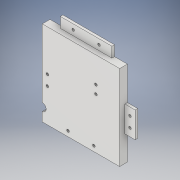
# Autodesk Inventor part: CP007
Saved by Autodesk Inventor 2017 SP1 (Build 210196100, 196)
## iProperties
Created: 2017-05-15
Part Number: CP007
Material: ABS Plastic
Document SubType Name: Modeling
Designer: zallen
Density: 1.06 g/cm^3
Appearance: Smooth - White
Mass: 391.263 g
Surface Area: 662.381 cm^2
Volume: 369.116 cm^3
Author: zallen
Autodesk Inventor part; units mm, degrees
ref_plane "YZ Plane" through (0, 0, 0) normal (1, 0, 0) x (0, 1, 0)
ref_plane "XZ Plane" through (0, 0, 0) normal (0, 1, 0) x (-1, 0, 0)
ref_plane "XY Plane" through (0, 0, 0) normal (0, 0, 1) x (1, 0, 0)
sketch "Sketch1" plane through (0, 0, 0) normal (0, 0, 1) x (1, 0, 0)
  line L0 (0, 0) -> (150, 0)
  line L1 (150, 0) -> (150, 164.5751)
  line L2 (150, 164.5751) -> (0, 164.5751)
  line L3 (0, 164.5751) -> (0, 0)
  dimension "d0" = 150
  dimension "d1" = 164.5751
  constraints: 8 end point, 2 parallel, 1 horizontal, 1 perpendicular
  measures "d0" distance of L2.end L1.end
  measures "d1" distance of L1.end L0.end
extrude "Extrusion1" add sketch "Sketch1" along normal blind 15
sketch "Sketch7" plane through (0, 0, 0) normal (0, 0, -1) x (-1, 0, 0)
  line L0 (-20, 50) -> (0, 50)
  line L1 (0, 50) -> (0, 100)
  line L2 (0, 100) -> (-20, 100)
  line L3 (-20, 100) -> (-20, 50)
  line L4 (0, 164.5751) -> (0, 0) projected
  dimension "d27" = 20
  dimension "d28" = 50
  dimension "d96" = 50
  constraints: 8 end point, 2 parallel, 1 horizontal, 1 perpendicular, 1 point on line
  measures "d27" distance of L2.end L1.end
  measures "d28" distance of L1.end L0.end
  measures "d96" distance of L0.end L4.end
extrude "Extrusion7" cut sketch "Sketch7" against normal blind 5
sketch "Sketch8" plane through (0, 0, 0) normal (0, 0, -1) x (-1, 0, 0)
  line L0 (-150, 164.5751) -> (0, 164.5751) projected
  line L1 (-25, 164.5751) -> (-125, 164.5751)
  line L2 (-125, 164.5751) -> (-125, 184.5751)
  line L3 (-125, 184.5751) -> (-25, 184.5751)
  line L4 (-25, 184.5751) -> (-25, 164.5751)
  point P0 (0, 0)
  dimension "d37" = 100
  dimension "d38" = 20
  dimension "d126" = 25
  constraints: 8 end point, 2 parallel, 1 horizontal, 1 perpendicular, 1 point on line
  measures "d37" distance of L2.end L3.end
  measures "d38" distance of L1.end L2.end
  measures "d126" distance from line of point (0, 0) L4
extrude "Extrusion8" add sketch "Sketch8" against normal blind 5
sketch "Sketch9" plane through (0, 0, 0) normal (0, 0, -1) x (-1, 0, 0)
  circle A0 centre (-50, 174.5751) radius 2.5
  circle A1 centre (-100, 174.5751) radius 2.5
  line L0 (-125, 184.5751) -> (-25, 184.5751) projected
  line L1 (0, 100) -> (0, 50) projected
  line L2 (0, 25) -> (20, 25) projected
  line L3 (20, 75) -> (0, 75) projected
  point P0 (0, 0)
  dimension "d44" = 5
  dimension "d45" = 5
  dimension "d46" = 10
  constraints: 2 centre point, 1 horizontal alignment
  measures "d44" diameter of A0
  measures "d45" diameter of A1
  measures "d46" distance from line of L0 A0.centre
extrude "Extrusion9" cut sketch "Sketch9" against normal through all
thread "Thread1" size "M5x0.8" class "6H" standard "ANSI Metric M Profile" full length
thread "Thread2" size "M5x0.8" class "6H" standard "ANSI Metric M Profile" full length
sketch "Sketch12" plane through (0, 0, 0) normal (0, 0, -1) x (-1, 0, 0)
  line L0 (0, 0) -> (-150, 0) projected
  line L1 (-25, 0) -> (-125, 0)
  line L2 (-125, 0) -> (-125, 20)
  line L3 (-125, 20) -> (-25, 20)
  line L4 (-25, 20) -> (-25, 0)
  dimension "d79" = 100
  dimension "d80" = 20
  dimension "d81" = 25
  constraints: 8 end point, 2 parallel, 1 horizontal, 1 perpendicular, 1 point on line
  measures "d79" distance of L2.end L3.end
  measures "d80" distance of L1.end L2.end
  measures "d81" distance from line of L0.start L4
extrude "Extrusion12" cut sketch "Sketch12" against normal blind 5
sketch "Sketch13" plane through (0, 0, 5) normal (0, 0, -1) x (-1, 0, 0)
  circle A0 centre (-50, 10) radius 2.5
  circle A1 centre (-100, 10) radius 2.5
  line L0 (-25, 20) -> (-25, 0) projected
  line L1 (-125, 0) -> (-125, 20) projected
  line L2 (-125, 20) -> (-25, 20) projected
  point P0 (0, 0)
  dimension "d84" = 5
  dimension "d85" = 5
  dimension "d86" = 25
  dimension "d87" = 25
  dimension "d88" = 10
  dimension "d89" = 10
  constraints: 2 centre point
  measures "d84" diameter of A0
  measures "d85" diameter of A1
  measures "d86" distance from line of A0.centre L0
  measures "d87" distance from line of L1 A1.centre
  measures "d88" distance from line of L2 A0.centre
  measures "d89" distance from line of L2 A1.centre
extrude "Extrusion13" cut sketch "Sketch13" against normal through all
thread "Thread9" size "M5x0.8" class "6H" standard "ANSI Metric M Profile" full length
thread "Thread10" size "M5x0.8" class "6H" standard "ANSI Metric M Profile" full length
sketch "Sketch14" plane through (0, 0, 5) normal (0, 0, -1) x (-1, 0, 0)
  circle A0 centre (-10, 65) radius 2.5
  circle A1 centre (-10, 85) radius 2.5
  line L0 (-20, 50) -> (-20, 100) projected
  line L1 (0, 50) -> (-20, 50) projected
  line L2 (-20, 100) -> (0, 100) projected
  point P0 (0, 0)
  dimension "d97" = 5
  dimension "d98" = 5
  dimension "d99" = 10
  dimension "d100" = 15
  dimension "d101" = 15
  dimension "d102" = 10
  constraints: 2 centre point
  measures "d97" diameter of A0
  measures "d98" diameter of A1
  measures "d99" distance from line of L0 A0.centre
  measures "d100" distance from line of L1 A0.centre
  measures "d101" distance from line of L2 A1.centre
  measures "d102" distance from line of L0 A1.centre
extrude "Extrusion14" cut sketch "Sketch14" against normal through all
thread "Thread11" size "M5x0.8" class "6H" standard "ANSI Metric M Profile" full length
thread "Thread12" size "M5x0.8" class "6H" standard "ANSI Metric M Profile" full length
sketch "Sketch15" plane through (0, 0, 0) normal (0, 0, -1) x (-1, 0, 0)
  line L0 (-150, 0) -> (-150, 164.5751) projected
  line L1 (-150, 50) -> (-170, 50)
  line L2 (-170, 50) -> (-170, 100)
  line L3 (-170, 100) -> (-150, 100)
  line L4 (-150, 100) -> (-150, 50)
  point P0 (0, 0)
  dimension "d109" = 20
  dimension "d110" = 50
  dimension "d111" = 50
  constraints: 8 end point, 2 parallel, 1 horizontal, 1 perpendicular, 1 point on line
  measures "d109" distance of L2.end L3.end
  measures "d110" distance of L1.end L2.end
  measures "d111" distance of L0.start L1.start
extrude "Extrusion15" add sketch "Sketch15" against normal blind 5
sketch "Sketch16" plane through (0, 0, 0) normal (0, 0, -1) x (-1, 0, 0)
  circle A0 centre (-160, 65) radius 2.5
  circle A1 centre (-160, 85) radius 2.5
  line L0 (-170, 50) -> (-170, 100) projected
  line L1 (-150, 50) -> (-170, 50) projected
  line L2 (-170, 100) -> (-150, 100) projected
  point P0 (0, 0)
  dimension "d114" = 5
  dimension "d115" = 5
  dimension "d116" = 10
  dimension "d117" = 10
  dimension "d118" = 15
  dimension "d119" = 15
  constraints: 2 centre point
  measures "d114" diameter of A0
  measures "d115" diameter of A1
  measures "d116" distance from line of L0 A0.centre
  measures "d117" distance from line of L0 A1.centre
  measures "d118" distance from line of L1 A0.centre
  measures "d119" distance from line of L2 A1.centre
extrude "Extrusion16" cut sketch "Sketch16" against normal through all
thread "Thread13" size "M5x0.8" class "6H" standard "ANSI Metric M Profile" full length
thread "Thread14" size "M5x0.8" class "6H" standard "ANSI Metric M Profile" full length
sketch "Sketch17" plane through (0, 0, 0) normal (0, 0, -1) x (-1, 0, 0)
  circle A0 centre (-104, 98.5751) radius 2.5
  circle A1 centre (-104, 114.5751) radius 2.5
  line L0 (-150, 0) -> (-150, 50) projected
  line L1 (-150, 164.5751) -> (0, 164.5751) projected
  line L2 (0, 164.5751) -> (0, 0) projected
  dimension "d127" = 5
  dimension "d128" = 5
  dimension "d130" = 16
  dimension "d145" = 50
  dimension "d146" = 104
  constraints: 2 centre point, 1 vertical alignment
  measures "d127" diameter of A0
  measures "d128" diameter of A1
  measures "d130" distance of A1.centre A0.centre
  measures "d145" distance from line of L1 A1.centre
  measures "d146" distance from line of L2 A0.centre
extrude "Extrusion17" cut sketch "Sketch17" against normal through all
thread "Thread17" size "M5x0.8" class "6H" standard "ANSI Metric M Profile" full length
thread "Thread18" size "M5x0.8" class "6H" standard "ANSI Metric M Profile" full length
sketch "Sketch18" plane through (0, 0, 0) normal (0, 0, -1) x (-1, 0, 0)
  line L0 (0, 50) -> (0, 0) projected
  circle A0 centre (0, 25) radius 7.5
  dimension "d142" = 15
  constraints: 1 centre point, 1 midpoint
  measures "d142" diameter of A0
extrude "Extrusion18" cut sketch "Sketch18" against normal through all
body "Solid1"
